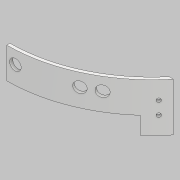
# Autodesk Inventor part: CW007
Saved by Autodesk Inventor 2017 (Build 210142000, 142)
## iProperties
Created: 2017-05-25
Part Number: CW007
Material: ABS Plastic
Document SubType Name: Modeling
Designer: zallen
Density: 1.06 g/cm^3
Appearance: CR White
Author: zallen
Autodesk Inventor part; units mm, degrees
sketch "Sketch1" plane through (0, 0, 0) normal (0, 0, 1) x (1, 0, 0)
  circle A0 centre (0, 225) radius 225 construction
  circle A1 centre (0, 225) radius 220 construction
  arc A2 (0, 0) -> (175, 83.5786) centre (0, 225) ccw
  line L0 (175, 83.5786) -> (168.523, 83.5786)
  line L1 (0, 0) -> (0, 5)
  arc A3 (0, 5) -> (168.523, 83.5786) centre (0, 225) ccw
  dimension "d0" = 450
  dimension "d1" = 5
  dimension "d2" = 175
  constraints: 8 point on circle, 4 centre point, 4 end point, 3 concentric, 1 horizontal, 1 vertical, 1 vertical alignment
  measures "d0" diameter of A0
  measures "d1" radial gap between concentric circles of A0 A1
  measures "d2" horizontal distance of L0.start L1.start
extrude "Extrusion1" add sketch "Sketch1" along normal blind 75
ref_plane "Work Plane1" through (0, 0, 0) normal (0, -1, 0) x (1, 0, 0)
sketch "Sketch2" plane through (0, 0, 0) normal (0, -1, 0) x (1, 0, 0)
  line L0 (0, 0) -> (150, 0)
  line L1 (150, 0) -> (150, 27)
  line L2 (150, 27) -> (0, 27)
  line L3 (0, 27) -> (0, 0)
  line L4 (0, 0) -> (175, 0) projected
  line L5 (175, 0) -> (175, 75) projected
  line L6 (0, 75) -> (175, 75) projected
  line L7 (0, 0) -> (0, 75) projected
  dimension "d5" = 27
  dimension "d6" = 25
  constraints: 8 end point, 2 parallel, 1 horizontal, 1 perpendicular
  measures "d5" distance of L1.end L0.end
  measures "d6" distance between parallel lines of L5 L1
extrude "Extrusion2" cut sketch "Sketch2" against normal through all contours L3 L2 L1 L0
ref_plane "Work Plane2" through (175, 83.5786, 0) normal (0.7778, -0.6285, 0) x (0.6285, 0.7778, 0)
sketch "Sketch3" plane through (175, 83.5786, 0) normal (0.7778, -0.6285, 0) x (0.6285, 0.7778, 0)
  circle A0 centre (-16, 47.5) radius 3
  circle A1 centre (-16, 27.5) radius 3
  line L0 (0, 0) -> (0, 75) projected
  line L1 (-36.1564, 27) -> (-36.1564, 0) projected
  line L2 (-36.1564, 0) -> (0, 0) projected
  line L3 (0, 0) -> (0, 75) projected
  line L4 (-175, 75) -> (0, 75) projected
  line L5 (-175, 27) -> (-175, 75) projected
  line L6 (-175, 27) -> (-36.1564, 27) projected
  point P0 (-175, 0)
  dimension "d9" = 6
  dimension "d10" = 6
  dimension "d11" = 16
  dimension "d12" = 27.5
  dimension "d13" = 20
  constraints: 2 centre point, 1 vertical alignment
  measures "d9" diameter of A0
  measures "d10" diameter of A1
  measures "d11" distance from line of L0 A1.centre
  measures "d12" distance from line of L2 A1.centre
  measures "d13" distance of A1.centre A0.centre
extrude "Extrusion3" cut sketch "Sketch3" against normal through all contours A0 | A1
sketch "Sketch4" plane through (0, 0, 0) normal (0, -1, 0) x (1, 0, 0)
  circle A0 centre (13, 55) radius 8.5
  line L0 (0, 27) -> (0, 75) projected
  line L1 (175, 75) -> (0, 75) projected
  point P0 (0, 0)
  dimension "d16" = 17
  dimension "d17" = 13
  dimension "d18" = 20
  constraints: 1 centre point
  measures "d16" diameter of A0
  measures "d17" distance from line of A0.centre L0
  measures "d18" distance from line of L1 A0.centre
extrude "Extrusion4" cut sketch "Sketch4" along normal through all both and the other way through all
ref_plane "Work Plane3" through (175, 83.5786, 75) normal (0.431, -0.9024, 0) x (-0.9024, -0.431, 0)
sketch "Sketch6" plane through (175, 83.5786, 75) normal (0.431, -0.9024, 0) x (-0.9024, -0.431, 0)
  circle A0 centre (101, 20) radius 8.5
  circle A1 centre (75, 20) radius 8.5
  line L0 (191.7792, 0) -> (5.8446, 0) projected
  point P0 (193.934, 75)
  point P1 (0, 0)
  dimension "d26" = 17
  dimension "d27" = 17
  dimension "d28" = 26
  dimension "d29" = 20
  dimension "d30" = 75
  constraints: 2 centre point, 1 horizontal alignment
  measures "d26" diameter of A0
  measures "d27" diameter of A1
  measures "d28" distance of A1.centre A0.centre
  measures "d29" distance from line of L0 A1.centre
  measures "d30" horizontal distance of point (0, 0) A1.centre
extrude "Extrusion5" cut sketch "Sketch6" along normal through all
body "Solid1"
